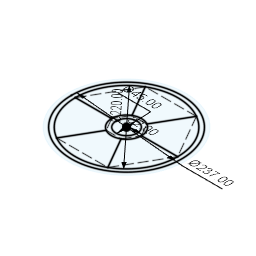
RadioactiveCAM (Autodesk Fusion 360 design; units mm, degrees)
Autodesk Fusion 360 part; units mm, degrees
sketch "Sketch1" plane through (0, 0, 0) normal (0, 0, 1) x (1, 0, 0)
  circle A0 centre (0, 0) radius 127
  dimension "d1" = 254
  constraint coincident A0.centre origin
  measures "d1" diameter of A0
extrude "Extrude1" add sketch "Sketch1" along normal blind 15.5
sketch "Sketch2" plane through (0, 0, 15.5) normal (0, 0, 1) x (-1, 0, 0)
  circle A0 centre (0, 0) radius 127
  circle A1 centre (0, 0) radius 22.5
  line L0 (-32, 0) -> (-16, -27.7128) construction
  line L1 (-16, -27.7128) -> (16, -27.7128) construction
  line L2 (16, -27.7128) -> (32, 0) construction
  line L3 (32, 0) -> (16, 27.7128) construction
  line L4 (16, 27.7128) -> (-16, 27.7128) construction
  line L5 (-16, 27.7128) -> (-32, 0) construction
  circle A2 centre (0, 0) radius 110
  line L6 (-32, 0) -> (-110, 0)
  line L7 (32, 0) -> (110, 0)
  line L8 (-16, -27.7128) -> (-55, -95.2628)
  line L9 (16, -27.7128) -> (55, -95.2628)
  line L10 (-55, -95.2628) -> (-110, 0) construction
  line L11 (55, -95.2628) -> (110, 0) construction
  line L12 (-16, 27.7128) -> (-55, 95.2628)
  line L13 (16, 27.7128) -> (55, 95.2628)
  line L14 (55, 95.2628) -> (-55, 95.2628) construction
  line L15 (-110, 0) -> (-55, 95.2628) construction
  line L16 (-55, -95.2628) -> (55, -95.2628) construction
  circle A3 centre (0, 0) radius 32
  circle A4 centre (0, 0) radius 118.5
  dimension "d4" = 45
  dimension "d5" = 32
  dimension "d6" = 220
  dimension "d7" = 237
  constraint concentric A0 A1
  constraint coincident A0.centre A1.centre
  constraint horizontal L4
  constraint concentric A0 A2
  constraint coincident A2 L6.end
  constraint horizontal L6
  constraint coincident A2 L7.end
  constraint horizontal L7
  constraint coincident A2 L8.end
  constraint coincident A2 L9.end
  constraint coincident A2 L12.end
  constraint coincident A2 L13.end
  constraint equal L10 L11
  constraint equal L10 L14
  constraint horizontal L14
  constraint equal L15 L16
  constraint concentric A1 A3
  constraint coincident L0.end A3
  constraint concentric A3 A4
  measures "d4" diameter of A1
  measures "d5" distance of L0.start A0.centre
  measures "d6" diameter of A2
  measures "d7" diameter of A4
extrude "Extrude3" [suppressed]
